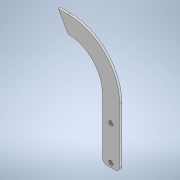
# Autodesk Inventor part: garrita
Saved by Autodesk Inventor 2022 (Build 260153000, 153)
## iProperties
Created: 2022-10-14
Part Number: garrita
Material: Generic
Document SubType Name: Modeling
Designer: Usuario
Density: 1 g/cm^3
Appearance: Default
Author: Usuario
Autodesk Inventor part; units mm, degrees
ref_plane "YZ Plane" through (0, 0, 0) normal (1, 0, 0) x (0, 1, 0)
ref_plane "XZ Plane" through (0, 0, 0) normal (0, 1, 0) x (-1, 0, 0)
ref_plane "XY Plane" through (0, 0, 0) normal (0, 0, 1) x (1, 0, 0)
sketch "Sketch1" plane through (0, 0, 0) normal (0, 0, 1) x (1, 0, 0)
  line L0 (20, 50) -> (20, -50)
  line L1 (10, -60) -> (-10, -60)
  line L2 (-20, -50) -> (-20, 50)
  arc A0 (10, -60) -> (20, -50) centre (10, -50) ccw
  arc A1 (-20, -50) -> (-10, -60) centre (-10, -50) ccw
  line L3 (-20, 80) -> (-20, 50)
  line L4 (20, 80) -> (20, 50)
  line L5 (-20, 80) -> (-100, 80) construction
  arc A2 (-20, 80) -> (-100, 160) centre (-100, 80) ccw
  arc A3 (20, 80) -> (-100, 200) centre (-100, 80) ccw
  line L6 (-100, 160) -> (-123.094, 200)
  line L7 (-100, 160) -> (-53.812, 160) construction
  line L8 (-123.094, 200) -> (-100, 200)
  point P0 (0, 0)
  point P1 (20, 0)
  point P2 (0, 80)
  dimension "d1" = 40
  dimension "d11" = 80
  dimension "d12" = 140
  dimension "d19" = 120
  constraints: 18 end point, 8 point on circle, 4 centre point, 4 tangent, 3 horizontal, 2 coincident, 1 equal length, 1 horizontal alignment, 1 midpoint, 1 parallel, 1 vertical alignment
  measures "d1" distance between parallel lines of L0 L2
  measures "d11" distance of L3.start L5.end
  measures "d12" distance from line of L1 point (0, 80)
  measures "d19" angle of L7 L6
extrude "Extrusion1" add sketch "Sketch1" along normal blind 5
sketch "Sketch3" plane through (0, 0, 5) normal (0, 0, 1) x (1, 0, 0)
  circle A0 centre (0, -50) radius 5
  line L0 (-10, -60) -> (10, -60) projected
  circle A1 centre (0, 30) radius 5
  point P0 (0, 0)
  dimension "d13" = 10
  dimension "d14" = 10
  dimension "d15" = 10
  dimension "d16" = 80
  constraints: 2 centre point
  measures "d13" diameter of A0
  measures "d14" distance from line of L0 A0.centre
  measures "d15" diameter of A1
  measures "d16" distance of A0.centre A1.centre
extrude "Extrusion3" cut sketch "Sketch3" against normal up to surface (5 mm away)
equation "\"d17\" = d13"
body "Solid1"
